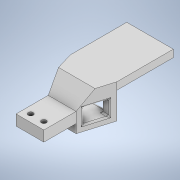
# Autodesk Inventor part: Finger_v2
Saved by Autodesk Inventor 2022 (Build 260153000, 153)
## iProperties
Created: 2021-09-24
Part Number: Finger_v2
Material: Generic
Document SubType Name: Modeling
Designer: kylem
Density: 1 g/cm^3
Appearance: Default
Author: kylem
Autodesk Inventor part; units mm, degrees
ref_plane "YZ Plane" through (0, 0, 0) normal (1, 0, 0) x (0, 1, 0)
ref_plane "XZ Plane" through (0, 0, 0) normal (0, 1, 0) x (-1, 0, 0)
sketch "Sketch2" plane through (0, 0, 0) normal (0, 1, 0) x (-1, 0, 0)
  line L0 (0, 0) -> (19, 0)
  line L1 (19, 0) -> (19, 22)
  line L2 (19, 22) -> (0, 22)
  line L3 (0, 22) -> (0, 0)
  line L4 (19, 22) -> (14, 22)
  line L5 (14, 22) -> (14, 17)
  line L6 (14, 17) -> (19, 17)
  line L7 (19, 17) -> (19, 22)
  line L8 (0, 22) -> (5, 22)
  line L9 (5, 22) -> (5, 17)
  line L10 (5, 17) -> (0, 17)
  line L11 (0, 17) -> (0, 22)
  circle A0 centre (14, 17) radius 1.7
  circle A1 centre (5, 17) radius 1.7
  dimension "d0" = 19
  dimension "d1" = 22
  dimension "d2" = 5
  dimension "d3" = 5
  dimension "d4" = 5
  dimension "d5" = 5
  dimension "d6" = 3.4
  dimension "d7" = 3.4
  constraints: 24 end point, 6 parallel, 3 horizontal, 3 perpendicular, 2 centre point, 2 coincident
  measures "d0" distance of L2.end L1.end
  measures "d1" distance of L1.end L0.end
  measures "d2" distance of L6.end L5.end
  measures "d3" distance of L5.end L4.end
  measures "d4" distance of L9.end L10.end
  measures "d5" distance of L8.end L9.end
  measures "d6" diameter of A0
  measures "d7" diameter of A1
extrude "Extrusion1" add sketch "Sketch2" along normal blind 17.2 contours L3 L10 A1 L9 L2 L5 A0 L6 L1 L0 | L3 L2 L9 A1 L10 | L6 A0 L5 L2 L1
sketch "Sketch4" plane through (0, 0, 22) normal (1, 0, 0) x (0, 0, -1)
  line L0 (0, 0) -> (17.2, 0)
  line L1 (17.2, 0) -> (-6, 0)
  line L2 (-6, 0) -> (-6, -60)
  line L3 (-6, -60) -> (17.2, -60)
  line L4 (17.2, -60) -> (17.2, 0)
  line L5 (0, 0) -> (17.2, 0)
  line L6 (17.2, 0) -> (-6, 0)
  line L7 (-6, 0) -> (-6, -60)
  line L8 (-6, -60) -> (17.2, -60)
  line L9 (17.2, -60) -> (17.2, 0)
  line L10 (0, 0) -> (22, 0) projected
  line L11 (22, 0) -> (22, -6)
  line L12 (22, -6) -> (82, -6)
  line L13 (82, -6) -> (82, 17.2)
  line L14 (82, 17.2) -> (22, 17.2)
  line L15 (22, 17.2) -> (22, -6)
  point P0 (0, 22)
  point P1 (0, 22)
  dimension "d15" = 23.2
  dimension "d16" = 60
  dimension "d17" = 23.2
  dimension "d18" = 60
  dimension "d19" = 6
  dimension "d20" = 60
  dimension "d21" = 23.2
  constraints: 30 end point, 6 parallel, 3 horizontal, 3 perpendicular, 1 vertical
  measures "d15" distance of L3.end L2.end
  measures "d16" distance of L2.end L1.end
  measures "d17" distance of L8.end L7.end
  measures "d18" distance of L7.end L6.end
  measures "d19" distance of L10.end L11.end
  measures "d20" distance of L14.end L13.end
  measures "d21" distance of L13.end L12.end
extrude "Extrusion2" add sketch "Sketch4" against normal blind 19 contours L15 L14 L13 L12 L11
sketch "Sketch5" plane through (0, -6, -60) normal (0, -1, 0) x (1, 0, 0)
  line L0 (0, 82) -> (0, 0) projected
  line L1 (-19, 82) -> (-19, 0) projected
  line L2 (0, 0) -> (-19, 0)
  line L3 (-19, 0) -> (-19, 38.5)
  line L4 (-19, 38.5) -> (0, 38.5)
  line L5 (0, 38.5) -> (0, 0)
  point P0 (0, 60)
  dimension "d24" = 38.5
  constraints: 8 end point, 2 parallel, 1 horizontal, 1 perpendicular, 1 point on line
  measures "d24" distance of L2.end L3.end
extrude "Extrusion3" cut sketch "Sketch5" against normal blind 18.2
sketch "Sketch6" plane through (0, 17.2, 0) normal (0, 1, 0) x (1, 0, 0)
  line L0 (0, -22) -> (0, 0) projected
  line L1 (-19, 21.5) -> (-19, 0) projected
  line L2 (0, -22) -> (-19, -22)
  line L3 (-19, -22) -> (-19, 0)
  line L4 (-19, 0) -> (0, 0)
  line L5 (0, 0) -> (0, -22)
  dimension "d27" = 22
  constraints: 8 end point, 2 parallel, 1 horizontal, 1 perpendicular
  measures "d27" distance of L2.end L1.end
extrude "Extrusion4" cut sketch "Sketch6" against normal blind 10
sketch "Sketch7" plane through (0, 17.2, 0) normal (0, 1, 0) x (1, 0, 0)
  line L0 (0, -22) -> (0, 0) projected
  line L1 (0, 0) -> (-19, 0) projected
  line L2 (0, 0) -> (-19, 0)
  line L3 (-9.5, 0) -> (6.4, 0)
  line L4 (6.4, 0) -> (6.4, 21.5)
  line L5 (0, 0) -> (0, 21.5) projected
  line L6 (6.4, 21.5) -> (0, 21.5)
  line L7 (0, 21.5) -> (0, 0)
  line L8 (0, 0) -> (6.4, 0)
  line L9 (6.4, 0) -> (6.4, 21.5)
  line L10 (-19, 21.5) -> (-19, 0) projected
  line L11 (-9.5, 0) -> (-19, 0)
  line L12 (-19, 0) -> (-19, 21.5)
  line L13 (-19, 21.5) -> (-9.5, 21.5)
  line L14 (-9.5, 21.5) -> (-9.5, 0)
  line L15 (-9.5, 0) -> (-25.4, 0)
  line L16 (-25.4, 0) -> (-25.4, 21.5)
  line L17 (-25.4, 21.5) -> (-9.5, 21.5)
  line L18 (-9.5, 21.5) -> (-9.5, 0)
  line L19 (6.4, 21.5) -> (0, 0)
  line L20 (-25.4, 21.5) -> (-19, 0)
  dimension "d30" = 15.9
  dimension "d31" = 21.5
  dimension "d32" = 15.9
  constraints: 34 end point, 6 parallel, 4 horizontal, 3 perpendicular, 2 point on line, 1 midpoint, 1 vertical
  measures "d30" distance of L3.start L3.end
  measures "d31" distance of L3.end L4.end
  measures "d32" distance of L16.end L17.end
extrude "Extrusion5" add sketch "Sketch7" against normal blind 23.2 contours L20 L17 L10 | L5 L6 L19
sketch "Sketch8" plane through (0, 17.2, 0) normal (0, 1, 0) x (1, 0, 0)
  line L0 (6.4, 21.5) -> (0, 0) projected
  line L1 (0, 21.5) -> (0, 60) projected
  line L2 (6.4, 21.5) -> (0, 21.5)
  line L3 (0, 21.5) -> (0, 60)
  line L4 (0, 60) -> (6.4, 60)
  line L5 (6.4, 60) -> (6.4, 21.5)
  line L6 (-19, 60) -> (-19, 21.5) projected
  line L7 (-19, 0) -> (-25.4, 21.5) projected
  line L8 (-19, 60) -> (-25.4, 60)
  line L9 (-25.4, 60) -> (-25.4, 21.5)
  line L10 (-25.4, 21.5) -> (-19, 21.5)
  line L11 (-19, 21.5) -> (-19, 60)
  constraints: 16 end point, 4 parallel, 2 horizontal, 2 perpendicular
extrude "Extrusion6" add sketch "Sketch8" against normal blind 5
chamfer "Chamfer1" distance 10 angle 45 1 edges at (-9.5, 17.2, 0)
ref_plane "Work Plane1" through (-25.4, 8, -21.5) normal (0, -1, 0) x (1, 0, 0)
sketch "Sketch9" plane through (-25.4, 8, -21.5) normal (0, -1, 0) x (1, 0, 0)
  line L0 (38.5, 31.8) -> (31.8, 31.8)
  line L1 (38.5, 0) -> (31.8, 0)
  line L2 (31.8, 31.8) -> (31.8, 0)
  line L3 (31.8, 0) -> (31.8, 31.8)
  line L4 (15.9, 0) -> (26.3, 0)
  line L5 (26.3, 0) -> (5.5, 0)
  line L6 (5.5, 0) -> (5.5, -14)
  line L7 (5.5, -14) -> (35.0442, -19.2094)
  line L8 (26.3, 0) -> (26.3, -4)
  line L9 (26.3, -4) -> (36.3, -4)
  line L10 (35.0442, -19.2094) -> (36.3, -4)
  line L11 (15.9, 0) -> (15.9, 6.734)
  line L12 (31.8, -31.8) -> (31.8, 0)
  line L13 (31.8, 0) -> (31.8, -31.8)
  line L14 (5.5, 0) -> (5.5, 14)
  line L15 (5.5, 14) -> (35.0442, 19.2094)
  line L16 (26.3, 0) -> (26.3, 4)
  line L17 (26.3, 4) -> (36.3, 4)
  line L18 (35.0442, 19.2094) -> (36.3, 4)
  line L19 (15.9, 0) -> (15.9, -6.734)
  point P0 (25.4, 21.5)
  point P1 (-43.5, 6.4)
  point P2 (0, 5.5)
  point P3 (0, 26.3)
  point P4 (0, 4)
  point P5 (5.5, 0)
  point P6 (26.3, 0)
  point P7 (0, 18.6374)
  point P8 (15.9, 0)
  point P9 (31.8, 4)
  point P10 (31.8, 18.6374)
  dimension "d41" = 10.4
  dimension "d42" = 20.8
  dimension "d43" = 14
  dimension "d44" = 30
  dimension "d45" = 100
  dimension "d46" = 4
  dimension "d47" = 10
  dimension "d48" = 90
  constraints: 40 end point, 6 symmetric about line, 1 perpendicular, 1 vertical
  measures "d41" distance of L4.start L4.end
  measures "d42" distance of L4.end L5.end
  measures "d43" distance of L5.end L6.end
  measures "d44" distance of L6.end L7.end
  measures "d45" angle of L7 L6
  measures "d46" distance of L4.end L8.end
  measures "d47" distance of L8.end L9.end
  measures "d48" angle of L9 L8
extrude "Extrusion8" cut sketch "Sketch9" along normal blind 10 contours L2 L17 L16 L4 L5 L14 L15
fillet "Fillet5" radius 2 4 edges at (-19.9, 3, -21.5) (-9.5, 8, -21.5) (-9.5, -2, -21.5) (0.9, 3, -21.5)
fillet "Fillet6" radius 1 4 edges at (3.1691, -2, -10.646) (1.1288, 3, -3.7921) (3.1691, 8, -10.646) (5.2093, 3, -17.5)
fillet "Fillet7" radius 1 12 edges at (4.3163, 8.0104, -17.5) (5.0614, 8.4022, -17.6983) (2.533, 8, -17.5) (4.3163, -2.0104, -17.5) (5.0614, -2.4022, -17.6983) (2.533, -2, -17.5) (0.0801, -2, -3.9753) (0.7297, -2.2929, -3.478) (-9.938, -2, -5.7434) (0.0801, 8, -3.9753) (0.7297, 8.2929, -3.478) (-9.938, 8, -5.7434)
fillet "Fillet8" radius 1 4 edges at (1.4858, 8.5858, -20.9142) (0.9, 8, -18.5) (1.4858, -2.5858, -20.9142) (0.9, -2, -18.5)
body "Solid1"
